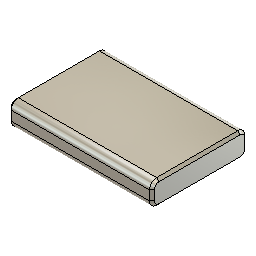
Design_1 (Autodesk Fusion 360 archive; units mm, degrees)
design "lipo"
Autodesk Fusion 360 part; units mm, degrees
sketch "Sketch1" plane through (0, 0, 0) normal (0, 1, 0) x (1, 0, 0)
  line L0 (-15, 10) -> (15, 10)
  line L1 (15, 10) -> (15, -10)
  line L2 (15, -10) -> (-15, -10)
  line L3 (-15, -10) -> (-15, 10)
  line L4 (-15, 10) -> (15, -10) construction
  line L5 (15, 10) -> (-15, -10) construction
  dimension "d1" = 30
  dimension "d2" = 20
  constraint perpendicular L0 L1
  constraint parallel L0 L2
  constraint parallel L1 L3
  constraint horizontal L0
  constraint coincident L4 origin
  constraint coincident L5 origin
  measures "d1" distance of L1.end L2.end
  measures "d2" distance of L0.end L1.end
extrude "Extrude1" add sketch "Sketch1" along normal blind 5
fillet "Fillet1" radius 1.5 4 edges at (0, 5, 10) (0, 0, 10) (0, 5, -10) (0, 0, -10)
chamfer "Chamfer1" distance 0.5 angle 45 16 edges at (-15, 2.5, 10) (-15, 0.4393, 9.5607) (-15, 0, 0) (-15, 0.4393, -9.5607) (-15, 2.5, -10) (-15, 4.5607, -9.5607) (-15, 5, 0) (-15, 4.5607, 9.5607) (15, 2.5, -10) (15, 0.4393, -9.5607) (15, 0, 0) (15, 0.4393, 9.5607) (15, 2.5, 10) (15, 4.5607, 9.5607) (15, 5, 0) (15, 4.5607, -9.5607)
